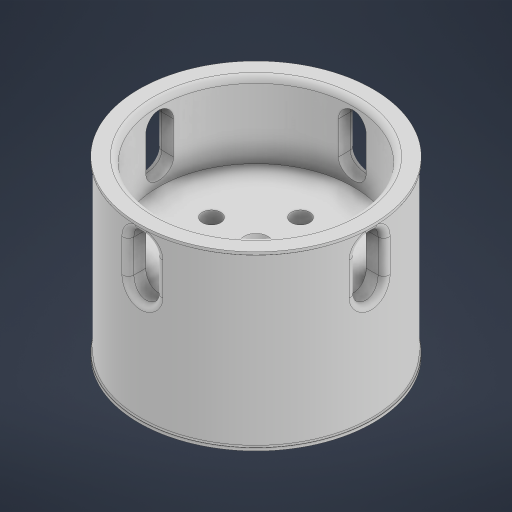
# Autodesk Inventor part: roda
Saved by Autodesk Inventor 2024.3 (Build 283343000, 343)
## iProperties
Created: 2025-06-15
Part Number: roda
Material: Generic
Document SubType Name: Modeling
Designer: Akbar Syihabuddin
Density: 1 g/cm^3
Appearance: Default
Author: Akbar Syihabuddin
Autodesk Inventor part; units mm, degrees
ref_plane "YZ Plane" through (0, 0, 0) normal (1, 0, 0) x (0, 1, 0)
ref_plane "XZ Plane" through (0, 0, 0) normal (0, 1, 0) x (-1, 0, 0)
ref_plane "XY Plane" through (0, 0, 0) normal (0, 0, 1) x (1, 0, 0)
sketch "Sketch1" plane through (0, 0, 0) normal (0, 1, 0) x (-1, 0, 0)
  circle A0 centre (0, 0) radius 20.75
  dimension "d0" = 41.5
  constraints: 1 centre point, 1 coincident
  measures "d0" diameter of A0
extrude "Extrusion1" add sketch "Sketch1" along normal blind 30
sketch "Sketch2" plane through (0, 30, 0) normal (0, 1, 0) x (1, 0, 0)
  circle A0 centre (0, 0) radius 17.5
  dimension "d3" = 35
  constraints: 1 centre point, 1 coincident
  measures "d3" diameter of A0
extrude "Extrusion2" cut sketch "Sketch2" against normal blind 13
sketch "Sketch3" plane through (0, 17, 0) normal (0, 1, 0) x (1, 0, 0)
  circle A0 centre (0, 0) radius 2
  circle A1 centre (-8, 0) radius 1.5
  circle A2 centre (-8, 0) radius 1.5
  circle A3 centre (0, -8) radius 1.5
  circle A4 centre (0, -8) radius 1.5
  circle A5 centre (8, 0) radius 1.5
  circle A6 centre (8, 0) radius 1.5
  circle A7 centre (0, 8) radius 1.5
  circle A8 centre (0, 8) radius 1.5
  circle A9 centre (0, 0) radius 11.0573
  constraints: 10 centre point, 8 coincident
extrude "Extrusion3" cut sketch "Sketch3" against normal blind 20 contours A0 | A1 | A3 | A5 | A7
sketch "Sketch4" plane through (0, 17, 0) normal (0, 1, 0) x (1, 0, 0)
  circle A0 centre (0, 0) radius 2 projected
  circle A1 centre (0, 0) radius 2.15
  circle A2 centre (0, -8) radius 1.5 projected
  circle A3 centre (0, -8) radius 1.65
  circle A4 centre (-8, 0) radius 1.5 projected
  circle A5 centre (-8, 0) radius 1.65
  circle A6 centre (0, 8) radius 1.5 projected
  circle A7 centre (0, 8) radius 1.65
  circle A8 centre (8, 0) radius 1.5 projected
  circle A9 centre (8, 0) radius 1.65
  dimension "d8" = 4.3
  dimension "d9" = 3.3
  dimension "d10" = 3.3
  dimension "d11" = 3.3
  dimension "d12" = 3.3
  constraints: 5 centre point, 5 coincident
  measures "d8" diameter of A1
  measures "d9" diameter of A3
  measures "d10" diameter of A5
  measures "d11" diameter of A7
  measures "d12" diameter of A9
extrude "Extrusion4" cut sketch "Sketch4" against normal blind 20 contours A0 | A1 | A3 | A4 | A5 | A6 | A7 | A8 | A9
sketch "Sketch5" plane through (0, 0, 0) normal (1, 0, 0) x (0, 1, 0)
  line L0 (17, 17.5) -> (17, -17.5) projected
  circle A0 centre (20.5076, 0) radius 2.5
  circle A1 centre (26.4365, 0) radius 2.5
  line L1 (20.5076, -2.5) -> (26.4365, -2.5)
  line L2 (26.4365, 2.5) -> (20.5076, 2.5)
  point P0 (0, 0)
  dimension "d15" = 5
  dimension "d16" = 5
  constraints: 4 end point, 4 point on circle, 3 tangent, 2 centre point, 1 horizontal
  measures "d15" diameter of A0
  measures "d16" diameter of A1
extrude "Extrusion5" cut sketch "Sketch5" along normal mid plane 400
pattern_circular "Circular Pattern1" count 4 over 360 about axis through (0, 17, 0) along (0, -1, 0) of "Extrusion5"
sketch "Sketch6" plane through (0, 30, 0) normal (0, 1, 0) x (1, 0, 0)
  circle A0 centre (0, 0) radius 17.5
  circle A1 centre (0, 0) radius 20.75
  circle A2 centre (0, 0) radius 21
  dimension "d22" = 42
  constraints: 3 centre point, 3 coincident
  measures "d22" diameter of A2
extrude "Extrusion6" add sketch "Sketch6" along normal blind 0.5 contours A0 | A1 | A2
extrude "Extrusion7" cut sketch "Sketch6" along normal blind 1 contours A0
sketch "Sketch7" plane through (0, 0, 0) normal (0, -1, 0) x (1, 0, 0)
  circle A0 centre (0, 0) radius 21
  circle A1 centre (0, 0) radius 17.5
  dimension "d28" = 42
  dimension "d29" = 35
  constraints: 2 centre point, 2 coincident
  measures "d28" diameter of A0
  measures "d29" diameter of A1
extrude "Extrusion8" add sketch "Sketch7" along normal blind 0.5
fillet "Fillet3" radius 0.2 2 edges at (20.75, 30, 0) (20.75, 0, 0)
fillet "Fillet4" radius 1 1 edges at (-17.5, 30.5, 0)
fillet "Fillet5" radius 1 5 edges at (-9.65, 0, 0) (-1.65, 0, 8) (-2.15, 0, 0) (-1.65, 0, -8) (6.35, 0, 0)
fillet "Fillet6" radius 1 14 edges at (2.5, 23.4721, -20.5988) (2.5, 23.4721, 20.5988) (0.3782, 28.9078, -20.7466) (0.3782, 28.9078, 20.7466) (-2.5, 23.4721, -20.5988) (-2.5, 23.4721, 20.5988) (0.0394, 18.008, -20.75) (0.0373, 18.0079, 20.75) (20.75, 28.9365, -0.0083) (20.5988, 23.4721, 2.5) (-20.5988, 23.4721, 2.5) (20.75, 18.0077, 0.0083) (20.5988, 23.4721, -2.5) (-20.5988, 23.4721, -2.5)
fillet "Fillet7" radius 1 1 edges at (-17.5, 0, 0)
body "Solid1"
